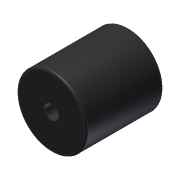
# Autodesk Inventor part: Conveyor_Roller_Middle
Saved by Autodesk Inventor 2012 (Build 160160000, 160)
## iProperties
Created: 2012-01-13
Part Number: Conveyor_Roller_Middle
Material: Rubber
Document SubType Name: Modeling
Designer: JesseK
Mass: 24.6622 g
Surface Area: 56.3194 cm^2
Volume: 26.5185 cm^3
Density: 0.93 g/cm^3
Author: JesseK
Autodesk Inventor part; units mm, degrees
ref_plane "YZ Plane" through (0, 0, 0) normal (1, 0, 0) x (0, 1, 0)
ref_plane "XZ Plane" through (0, 0, 0) normal (0, 1, 0) x (-1, 0, 0)
ref_plane "XY Plane" through (0, 0, 0) normal (0, 0, 1) x (1, 0, 0)
sketch "Sketch1" plane through (0, 0, 0) normal (0, 0, 1) x (1, 0, 0)
  circle A0 centre (0, 0) radius 15.875
  circle A1 centre (0, 0) radius 3.175
  dimension "d0" = 31.75
  dimension "d1" = 6.35
  constraints: 2 centre point, 2 coincident
  measures "d0" diameter of A0
  measures "d1" diameter of A1
extrude "Extrusion1" add sketch "Sketch1" along normal blind 34.925
fillet "Fillet1" radius 0.7937 2 edges at (-15.875, 0, 34.925) (-15.875, 0, 0)
body "Solid1"
